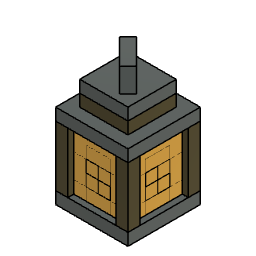
MinecraftMiniLaterne (Autodesk Fusion 360 design; units mm, degrees)
Autodesk Fusion 360 part; units mm, degrees
sketch "Skizze1" plane through (0, 0, 0) normal (0, 0, 1) x (1, 0, 0)
  line L0 (0, 0) -> (60, 0)
  line L1 (60, 0) -> (60, 60)
  line L2 (60, 60) -> (0, 60)
  line L3 (0, 60) -> (0, 0)
  line L4 (0, 0) -> (10, 0)
  line L5 (10, 0) -> (10, 10)
  line L6 (10, 10) -> (0, 10)
  line L7 (0, 10) -> (0, 0)
  line L8 (0, 60) -> (60, 0) construction
  line L9 (60, 60) -> (30, 30) construction
  line L10 (30, 30) -> (0, 0) construction
  line L11 (60, 0) -> (60, 10)
  line L12 (60, 10) -> (50, 10)
  line L13 (50, 10) -> (50, 0)
  line L14 (50, 0) -> (60, 0)
  line L15 (60, 60) -> (50, 60)
  line L16 (50, 60) -> (50, 50)
  line L17 (50, 50) -> (60, 50)
  line L18 (60, 50) -> (60, 60)
  line L19 (0, 60) -> (0, 50)
  line L20 (0, 50) -> (10, 50)
  line L21 (10, 50) -> (10, 60)
  line L22 (10, 60) -> (0, 60)
  line L23 (10, 50) -> (50, 50)
  line L24 (50, 50) -> (50, 10)
  line L25 (50, 10) -> (10, 10)
  line L26 (10, 10) -> (10, 50)
  line L27 (10, 10) -> (7, 10) construction
  line L28 (7, 10) -> (5, 10)
  line L29 (5, 10) -> (5, 50)
  line L30 (5, 50) -> (7, 50)
  line L31 (7, 50) -> (7, 10)
  line L32 (50, 5) -> (10, 5)
  line L33 (10, 5) -> (10, 7)
  line L34 (10, 7) -> (50, 7)
  line L35 (50, 7) -> (50, 5)
  line L36 (55, 50) -> (55, 10)
  line L37 (55, 10) -> (53, 10)
  line L38 (53, 10) -> (53, 50)
  line L39 (53, 50) -> (55, 50)
  line L40 (10, 55) -> (50, 55)
  line L41 (50, 55) -> (50, 53)
  line L42 (50, 53) -> (10, 53)
  line L43 (10, 53) -> (10, 55)
  line L44 (7, 10) -> (5, 10)
  line L45 (5, 10) -> (5, 8)
  line L46 (5, 8) -> (7, 8)
  line L47 (7, 8) -> (7, 10)
  line L48 (10, 7) -> (8, 7)
  line L49 (8, 7) -> (8, 5)
  line L50 (8, 5) -> (10, 5)
  line L51 (10, 5) -> (10, 7)
  line L52 (53, 10) -> (53, 8)
  line L53 (55, 8) -> (55, 10)
  line L54 (55, 10) -> (53, 10)
  line L55 (53, 8) -> (55, 8)
  line L56 (50, 7) -> (50, 5)
  line L57 (50, 5) -> (52, 5)
  line L58 (52, 7) -> (50, 7)
  line L59 (52, 5) -> (52, 7)
  line L60 (50, 53) -> (52, 53)
  line L61 (52, 55) -> (50, 55)
  line L62 (50, 55) -> (50, 53)
  line L63 (52, 53) -> (52, 55)
  line L64 (53, 50) -> (55, 50)
  line L65 (55, 50) -> (55, 52)
  line L66 (53, 52) -> (53, 50)
  line L67 (55, 52) -> (53, 52)
  line L68 (7, 50) -> (7, 52)
  line L69 (5, 52) -> (5, 50)
  line L70 (5, 50) -> (7, 50)
  line L71 (7, 52) -> (5, 52)
  line L72 (10, 53) -> (10, 55)
  line L73 (10, 55) -> (8, 55)
  line L74 (8, 53) -> (10, 53)
  line L75 (8, 55) -> (8, 53)
  line L76 (0, 10) -> (10, 0) construction
  line L77 (7, 3) -> (3, 3)
  line L78 (3, 3) -> (3, 7)
  line L79 (3, 7) -> (7, 7)
  line L80 (7, 7) -> (7, 3)
  line L81 (7, 3) -> (3, 7) construction
  line L82 (3, 3) -> (7, 7) construction
  line L83 (57, 7) -> (57, 3)
  line L84 (57, 3) -> (53, 3)
  line L85 (53, 7) -> (57, 7)
  line L86 (53, 3) -> (53, 7)
  line L87 (53, 57) -> (57, 57)
  line L88 (57, 57) -> (57, 53)
  line L89 (53, 53) -> (53, 57)
  line L90 (57, 53) -> (53, 53)
  line L91 (3, 53) -> (3, 57)
  line L92 (3, 57) -> (7, 57)
  line L93 (7, 53) -> (3, 53)
  line L94 (7, 57) -> (7, 53)
  line L95 (2.8, 7.2) -> (7.2, 7.2)
  line L96 (7.2, 7.2) -> (7.2, 2.8)
  line L97 (7.2, 2.8) -> (2.8, 2.8)
  line L98 (2.8, 2.8) -> (2.8, 7.2)
  line L99 (57.2, 2.8) -> (52.8, 2.8)
  line L100 (52.8, 2.8) -> (52.8, 7.2)
  line L101 (57.2, 7.2) -> (57.2, 2.8)
  line L102 (52.8, 7.2) -> (57.2, 7.2)
  line L103 (57.2, 57.2) -> (57.2, 52.8)
  line L104 (57.2, 52.8) -> (52.8, 52.8)
  line L105 (52.8, 57.2) -> (57.2, 57.2)
  line L106 (52.8, 52.8) -> (52.8, 57.2)
  line L107 (2.8, 57.2) -> (7.2, 57.2)
  line L108 (7.2, 57.2) -> (7.2, 52.8)
  line L109 (2.8, 52.8) -> (2.8, 57.2)
  line L110 (7.2, 52.8) -> (2.8, 52.8)
  point P0 (5, 5)
  dimension "d1" = 60
  dimension "d2" = 60
  dimension "d3" = 10
  dimension "d4" = 10
  dimension "d9" = 360
  dimension "d10" = 3
  dimension "d11" = 2
  dimension "d13" = 360
  dimension "d54" = 2
  dimension "d55" = 2
  dimension "d56" = 2
  dimension "d57" = 2
  dimension "d113" = 4
  dimension "d114" = 4
  dimension "d122" = -0.2
  constraint horizontal L0
  constraint vertical L1
  constraint horizontal L2
  constraint vertical L3
  constraint coincident L0.start L3.end
  constraint horizontal L4
  constraint vertical L5
  constraint horizontal L6
  constraint vertical L7
  constraint midpoint L8 L9.end
  constraint horizontal L23
  constraint vertical L24
  constraint horizontal L25
  constraint vertical L26
  constraint perpendicular L5 L27
  constraint horizontal L28
  constraint vertical L29
  constraint horizontal L30
  constraint vertical L31
  constraint coincident L20 L29.end
  constraint horizontal L44
  constraint vertical L45
  constraint horizontal L46
  constraint vertical L47
  constraint horizontal L48
  constraint vertical L49
  constraint horizontal L50
  constraint vertical L51
  constraint horizontal L77
  constraint perpendicular L77 L78
  constraint parallel L77 L79
  constraint parallel L78 L80
  constraint coincident L81 P0
  constraint coincident L82 P0
  constraint midpoint L76 P0
  measures "d1" distance of L0.start L0.end
  measures "d2" distance of L0.start L2.end
  measures "d3" distance of L0.start L4.end
  measures "d4" distance of L0.start L6.end
  measures "d10" distance of L5.end L27.end
  measures "d11" distance of L27.end L28.end
  measures "d54" distance of L27.end L46.end
  measures "d55" distance of L45.end L46.end
  measures "d56" distance of L33.end L48.end
  measures "d57" distance of L33.end L32.end
  measures "d113" distance of L78.end L79.end
  measures "d114" distance of L77.end L78.end
ref_plane "Arbeitsebene1" through (30, 0, 0) normal (1, 0, 0) x (0, 1, 0)
sketch "Skizze3" plane through (30, 0, 0) normal (1, 0, 0) x (0, 1, 0)
  line L0 (0, 0) -> (60, 0)
  line L1 (30, 0) -> (30, 100) construction
  point P0 (30, 0)
  dimension "d92" = 100
  constraint coincident P0 L1.start
  constraint perpendicular L0 L1
  measures "d92" distance of P0 L1.end
sketch "Skizze2" plane through (0, 0, 0) normal (1, 0, 0) x (0, 1, 0)
  line L0 (0, 0) -> (60, 0)
  line L1 (60, 0) -> (60, 10)
  line L2 (60, 10) -> (0, 10)
  line L3 (0, 10) -> (0, 0)
  line L4 (0, 10) -> (10, 10)
  line L5 (10, 10) -> (10, 60)
  line L6 (10, 60) -> (0, 60)
  line L7 (0, 60) -> (0, 10)
  line L8 (0, 60) -> (60, 60)
  line L9 (60, 60) -> (60, 70)
  line L10 (60, 70) -> (0, 70)
  line L11 (0, 70) -> (0, 60)
  line L12 (60, 10) -> (50, 10)
  line L13 (50, 10) -> (50, 60)
  line L14 (50, 60) -> (60, 60)
  line L15 (60, 60) -> (60, 10)
  line L16 (50, 60) -> (52, 60) construction
  line L17 (52, 60) -> (52, 62) construction
  line L18 (52, 62) -> (50, 62) construction
  line L19 (50, 62) -> (50, 60) construction
  line L20 (10, 10) -> (8, 10) construction
  line L21 (8, 10) -> (8, 8) construction
  line L22 (8, 8) -> (10, 8) construction
  line L23 (10, 8) -> (10, 10) construction
  line L24 (8, 8) -> (52, 8)
  line L25 (52, 8) -> (52, 62)
  line L26 (52, 62) -> (8, 62)
  line L27 (8, 62) -> (8, 8)
  line L28 (50, 10) -> (40, 10)
  line L29 (40, 10) -> (40, 20)
  line L30 (40, 20) -> (50, 20)
  line L31 (50, 20) -> (50, 10)
  line L32 (40, 20) -> (30, 20)
  line L33 (30, 20) -> (30, 30)
  line L34 (30, 30) -> (40, 30)
  line L35 (40, 30) -> (40, 20)
  line L36 (30, 20) -> (20, 20)
  line L37 (20, 20) -> (20, 10)
  line L38 (20, 10) -> (30, 10)
  line L39 (30, 10) -> (30, 20)
  line L40 (20, 20) -> (10, 20)
  line L41 (10, 20) -> (10, 30)
  line L42 (10, 30) -> (20, 30)
  line L43 (20, 30) -> (20, 20)
  line L44 (40, 30) -> (50, 30)
  line L45 (50, 30) -> (50, 40)
  line L46 (50, 40) -> (40, 40)
  line L47 (40, 40) -> (40, 30)
  line L48 (20, 30) -> (30, 30)
  line L49 (30, 30) -> (30, 40)
  line L50 (30, 40) -> (20, 40)
  line L51 (20, 40) -> (20, 30)
  line L52 (40, 40) -> (30, 40)
  line L53 (30, 40) -> (30, 50)
  line L54 (30, 50) -> (40, 50)
  line L55 (40, 50) -> (40, 40)
  line L56 (20, 40) -> (10, 40)
  line L57 (10, 40) -> (10, 50)
  line L58 (10, 50) -> (20, 50)
  line L59 (20, 50) -> (20, 40)
  line L60 (40, 50) -> (50, 50)
  line L61 (50, 50) -> (50, 60)
  line L62 (50, 60) -> (40, 60)
  line L63 (40, 60) -> (40, 50)
  line L64 (20, 50) -> (30, 50)
  line L65 (30, 50) -> (30, 60)
  line L66 (30, 60) -> (20, 60)
  line L67 (20, 60) -> (20, 50)
  line L68 (0, 70) -> (10, 70) construction
  line L69 (10, 70) -> (50, 70)
  line L70 (50, 70) -> (50, 80)
  line L71 (50, 80) -> (10, 80)
  line L72 (10, 80) -> (10, 70)
  line L73 (10, 80) -> (50, 80)
  line L74 (50, 80) -> (50, 90)
  line L75 (50, 90) -> (10, 90)
  line L76 (10, 90) -> (10, 80)
  line L77 (51.58, 61.58) -> (8.42, 61.58)
  line L78 (8.42, 61.58) -> (8.42, 8.42)
  line L79 (8.42, 8.42) -> (51.58, 8.42)
  line L80 (51.58, 8.42) -> (51.58, 61.58)
  dimension "d14" = 60
  dimension "d15" = 10
  dimension "d16" = 10
  dimension "d17" = 50
  dimension "d18" = 60
  dimension "d19" = 10
  dimension "d20" = 10
  dimension "d21" = 2
  dimension "d22" = 2
  dimension "d23" = 2
  dimension "d24" = 2
  dimension "d25" = 10
  dimension "d26" = 10
  dimension "d27" = 10
  dimension "d28" = 10
  dimension "d29" = 10
  dimension "d30" = 10
  dimension "d31" = 10
  dimension "d32" = 10
  dimension "d33" = 10
  dimension "d34" = 10
  dimension "d35" = 10
  dimension "d36" = 10
  dimension "d37" = 10
  dimension "d38" = 10
  dimension "d39" = 10
  dimension "d40" = 10
  dimension "d41" = 10
  dimension "d42" = 10
  dimension "d43" = 10
  dimension "d44" = 10
  dimension "d45" = 10
  dimension "d46" = 40
  dimension "d47" = 10
  dimension "d48" = 40
  dimension "d49" = 10
  dimension "d112" = -0.42
  constraint horizontal L0
  constraint vertical L1
  constraint horizontal L2
  constraint vertical L3
  constraint coincident L0.start L3.end
  constraint horizontal L4
  constraint vertical L5
  constraint horizontal L6
  constraint vertical L7
  constraint horizontal L8
  constraint vertical L9
  constraint horizontal L10
  constraint vertical L11
  constraint horizontal L12
  constraint vertical L13
  constraint horizontal L14
  constraint vertical L15
  constraint horizontal L16
  constraint vertical L17
  constraint horizontal L18
  constraint vertical L19
  constraint horizontal L20
  constraint vertical L21
  constraint horizontal L22
  constraint vertical L23
  constraint horizontal L24
  constraint vertical L25
  constraint horizontal L26
  constraint vertical L27
  constraint horizontal L28
  constraint vertical L29
  constraint horizontal L30
  constraint vertical L31
  constraint horizontal L32
  constraint vertical L33
  constraint horizontal L34
  constraint vertical L35
  constraint horizontal L36
  constraint vertical L37
  constraint horizontal L38
  constraint vertical L39
  constraint horizontal L40
  constraint vertical L41
  constraint horizontal L42
  constraint vertical L43
  constraint horizontal L44
  constraint vertical L45
  constraint horizontal L46
  constraint vertical L47
  constraint horizontal L48
  constraint vertical L49
  constraint horizontal L50
  constraint vertical L51
  constraint horizontal L52
  constraint vertical L53
  constraint horizontal L54
  constraint vertical L55
  constraint horizontal L56
  constraint vertical L57
  constraint horizontal L58
  constraint vertical L59
  constraint horizontal L60
  constraint vertical L61
  constraint horizontal L62
  constraint vertical L63
  constraint horizontal L64
  constraint vertical L65
  constraint horizontal L66
  constraint vertical L67
  constraint coincident L10 L68.end
  constraint horizontal L69
  constraint vertical L70
  constraint horizontal L71
  constraint vertical L72
  constraint horizontal L73
  constraint vertical L74
  constraint horizontal L75
  constraint vertical L76
  measures "d14" distance of L0.start L0.end
  measures "d15" distance of L0.start L2.end
  measures "d16" distance of L2.end L4.end
  measures "d17" distance of L2.end L6.end
  measures "d18" distance of L6.end L8.end
  measures "d19" distance of L6.end L10.end
  measures "d20" distance of L1.end L12.end
  measures "d21" distance of L13.end L16.end
  measures "d22" distance of L13.end L18.end
  measures "d23" distance of L4.end L20.end
  measures "d24" distance of L4.end L22.end
  measures "d25" distance of L12.end L28.end
  measures "d26" distance of L12.end L30.end
  measures "d27" distance of L29.end L32.end
  measures "d28" distance of L29.end L34.end
  measures "d29" distance of L32.end L36.end
  measures "d30" distance of L32.end L38.end
  measures "d31" distance of L36.end L40.end
  measures "d32" distance of L36.end L42.end
  measures "d33" distance of L34.end L44.end
  measures "d34" distance of L34.end L46.end
  measures "d35" distance of L42.end L33.end
  measures "d36" distance of L42.end L50.end
  measures "d37" distance of L46.end L49.end
  measures "d38" distance of L46.end L54.end
  measures "d39" distance of L50.end L56.end
  measures "d40" distance of L50.end L58.end
  measures "d41" distance of L54.end L60.end
  measures "d42" distance of L54.end L62.end
  measures "d43" distance of L58.end L53.end
  measures "d44" distance of L58.end L66.end
  measures "d45" distance of L10.end L68.end
  measures "d46" distance of L68.end L69.end
  measures "d47" distance of L68.end L71.end
  measures "d48" distance of L71.end L70.end
  measures "d49" distance of L71.end L75.end
extrude "Extrusion1" add sketch "Skizze1" along normal blind 10 contours L0 L3 L4 L5 L6 L7 L45 L46 L47 L48 L49 L50 | L0 L5 L13 L32 | L3 L6 L20 L29 | L0 L1 L11 L12 L13 L14 L52 L53 L55 L57 L58 L59 | L2 L3 L19 L20 L21 L22 L68 L69 L71 L73 L74 L75 | L5 L13 L25 L34 | L6 L20 L26 L31 | L1 L12 L17 L36 | L23 L24 L25 L26 | L2 L16 L21 L40 | L1 L2 L15 L16 L17 L18 L60 L61 L63 L65 L66 L67 | L12 L17 L24 L38 | L16 L21 L23 L42 | L77 L78 L79 L80 | L83 L84 L85 L86 | L87 L88 L89 L90 | L91 L92 L93 L94 | L95 L96 L97 L98 | L99 L100 L101 L102 | L103 L104 L105 L106 | L107 L108 L109 L110 makes body 1
extrude "Extrusion2" add sketch "Skizze1" along normal blind 8 contours L5 L33 L48 L49 L50 L51 | L5 L13 L32 L33 L34 L35 L51 L56 | L6 L20 L28 L29 L30 L31 L44 L70 | L6 L28 L44 L45 L46 L47 | L13 L35 L56 L57 L58 L59 | L20 L30 L68 L69 L70 L71 | L12 L37 L52 L53 L54 L55 | L12 L17 L36 L37 L38 L39 L54 L64 | L16 L21 L40 L41 L42 L43 L62 L72 | L21 L43 L72 L73 L74 L75 | L17 L39 L64 L65 L66 L67 | L16 L41 L60 L61 L62 L63 bodies 1
extrude "Extrusion3" add sketch "Skizze1" along normal blind 50 from surface at 10 separate body contours L0 L3 L4 L5 L6 L7 L45 L46 L47 L48 L49 L50 | L0 L1 L11 L12 L13 L14 L52 L53 L55 L57 L58 L59 | L2 L3 L19 L20 L21 L22 L68 L69 L71 L73 L74 L75 | L1 L2 L15 L16 L17 L18 L60 L61 L63 L65 L66 L67 | L77 L78 L79 L80 | L83 L84 L85 L86 | L87 L88 L89 L90 | L91 L92 L93 L94 | L95 L96 L97 L98 | L99 L100 L101 L102 | L103 L104 L105 L106 | L107 L108 L109 L110 makes body 2 at (0, 6.6667, 26.6667) makes body 3 at (6.6667, 60, 26.6667) makes body 4 at (60, 3.3333, 26.6667) makes body 5 at (56.6667, 60, 26.6667)
extrude "Extrusion18" add sketch "Skizze1" along normal blind 5 from surface at 60 contours L77 L78 L79 L80 | L83 L84 L85 L86 | L87 L88 L89 L90 | L91 L92 L93 L94 bodies 2 3 4 5
extrude "Extrusion4" add sketch "Skizze1" along normal blind 10 from surface at 60 separate body contours L0 L3 L4 L5 L6 L7 L45 L46 L47 L48 L49 L50 | L0 L5 L13 L32 | L3 L6 L20 L29 | L0 L1 L11 L12 L13 L14 L52 L53 L55 L57 L58 L59 | L2 L3 L19 L20 L21 L22 L68 L69 L71 L73 L74 L75 | L5 L13 L25 L34 | L6 L20 L26 L31 | L1 L12 L17 L36 | L23 L24 L25 L26 | L2 L16 L21 L40 | L1 L2 L15 L16 L17 L18 L60 L61 L63 L65 L66 L67 | L12 L17 L24 L38 | L16 L21 L23 L42 | L77 L78 L79 L80 | L83 L84 L85 L86 | L87 L88 L89 L90 | L91 L92 L93 L94 | L95 L96 L97 L98 | L99 L100 L101 L102 | L103 L104 L105 L106 | L107 L108 L109 L110 makes body 6
extrude "Extrusion19" cut sketch "Skizze1" along normal blind 7 from surface at 60 contours L77 L78 L79 L80 | L83 L84 L85 L86 | L87 L88 L89 L90 | L91 L92 L93 L94 | L95 L96 L97 L98 | L99 L100 L101 L102 | L103 L104 L105 L106 | L107 L108 L109 L110 bodies 6
extrude "Extrusion5" add sketch "Skizze1" against normal blind 8 from surface at 70 contours L5 L33 L48 L49 L50 L51 | L5 L13 L32 L33 L34 L35 L51 L56 | L6 L20 L28 L29 L30 L31 L44 L70 | L6 L28 L44 L45 L46 L47 | L13 L35 L56 L57 L58 L59 | L20 L30 L68 L69 L70 L71 | L12 L37 L52 L53 L54 L55 | L12 L17 L36 L37 L38 L39 L54 L64 | L16 L21 L40 L41 L42 L43 L62 L72 | L21 L43 L72 L73 L74 L75 | L17 L39 L64 L65 L66 L67 | L16 L41 L60 L61 L62 L63 bodies 6
extrude "Extrusion6" add sketch "Skizze2" along normal blind 40 from surface at 10 separate body contours L10 L69 L70 L71 L72 L73 makes body 7
extrude "Extrusion7" add sketch "Skizze2" along normal blind 40 from surface at 10 separate body contours L71 L73 L74 L75 L76 makes body 8
extrude "Extrusion8" add sketch "Skizze2" against normal blind 1.8 from surface at 7 separate body contours L2 L4 L5 L6 L8 L41 L57 L78 | L2 L4 L12 L28 L38 L78 L79 L80 | L2 L8 L12 L13 L14 L31 L45 L61 L80 | L6 L8 L14 L62 L66 L77 L78 L80 makes body 9
extrude "Extrusion9" add sketch "Skizze2" along normal blind 0.4 from surface at 5.2 separate body contours L32 L33 L34 L35 | L48 L49 L50 L51 makes body 10 at (5.2, 23.3333, 36.6667)
extrude "Extrusion10" add sketch "Skizze2" along normal blind 0.2 from surface at 5.2 contours L33 L36 L43 L48 | L34 L47 L49 L52 bodies 10
extrude "Extrusion11" add sketch "Skizze2" along normal blind 0.6 from surface at 5.2 contours L2 L36 L37 L38 L39 | L5 L40 L41 L42 L43 | L2 L29 L32 L39 | L13 L30 L35 L44 | L5 L42 L51 L56 | L13 L44 L45 L46 L47 | L50 L53 L59 L64 | L52 L53 L54 L55 bodies 9 10
extrude "Extrusion12" add sketch "Skizze2" along normal blind 0.8 from surface at 5.2 contours L2 L5 L37 L40 | L2 L13 L28 L29 L30 L31 | L5 L56 L57 L58 L59 | L8 L64 L65 L66 L67 | L8 L54 L63 L65 | L13 L46 L55 L60 bodies 9
extrude "Extrusion13" add sketch "Skizze2" along normal blind 1 from surface at 5.2 contours L5 L8 L58 L67 | L8 L13 L60 L61 L62 L63 bodies 9
pattern_circular "C-Anordnung1" count 4 over 360 about axis through (30, 30, 0) along (0, 0, 1) of bodies 9 makes body 11 at (22.8067, 5.2, 26.14) makes body 12 at (54.8, 22.8067, 26.14) makes body 13 at (37.1933, 54.8, 26.14)
sketch "Skizze4" plane through (0, 0, 90) normal (0, 0, 1) x (-1, 0, 0)
  line L0 (-10, -50) -> (-10, -10)
  line L1 (-10, -10) -> (-50, -10)
  line L2 (-50, -10) -> (-50, -50)
  line L3 (-50, -50) -> (-10, -50)
  line L4 (-50, -10) -> (-10, -50) construction
  line L5 (-10, -10) -> (-30, -30) construction
  line L6 (-30, -37.0711) -> (-37.0711, -30)
  line L7 (-37.0711, -30) -> (-30, -22.9289)
  line L8 (-30, -22.9289) -> (-22.9289, -30)
  line L9 (-22.9289, -30) -> (-30, -37.0711)
  line L10 (-30, -37.0711) -> (-30, -22.9289) construction
  line L11 (-37.0711, -30) -> (-22.9289, -30) construction
  line L12 (-30, -37.0711) -> (-22.9289, -30)
  line L13 (-22.9289, -30) -> (-15.8579, -37.0711)
  line L14 (-15.8579, -37.0711) -> (-22.9289, -44.1421)
  line L15 (-22.9289, -44.1421) -> (-30, -37.0711)
  line L16 (-37.0711, -30) -> (-30, -22.9289)
  line L17 (-30, -22.9289) -> (-37.0711, -15.8579)
  line L18 (-37.0711, -15.8579) -> (-44.1421, -22.9289)
  line L19 (-44.1421, -22.9289) -> (-37.0711, -30)
  point P0 (-30, -30)
  dimension "d95" = 10
  dimension "d96" = 10
  dimension "d97" = 10
  dimension "d98" = 10
  constraint coincident L1.end L2.start
  constraint coincident L0.start L3.end
  constraint coincident L0.end L1.start
  constraint midpoint L4 P0
  constraint perpendicular L6 L7
  constraint parallel L6 L8
  constraint parallel L7 L9
  constraint coincident L10 P0
  constraint coincident L11 P0
  constraint coincident P0 L5.end
  constraint perpendicular L12 L13
  constraint parallel L12 L14
  constraint parallel L13 L15
  constraint perpendicular L16 L17
  constraint parallel L16 L18
  constraint parallel L17 L19
  measures "d95" distance of L7.end L8.end
  measures "d96" distance of L6.end L7.end
  measures "d97" distance of L6.start L14.end
  measures "d98" distance of L6.end L18.end
extrude "Extrusion14" add sketch "Skizze4" along normal blind 10 separate body contours L9 L12 L13 L14 L15 | L7 L16 L17 L18 L19 makes body 14 at (39.4281, 27.643, 96.6667) makes body 15 at (18.2149, 39.4281, 93.3333)
extrude "Extrusion15" add sketch "Skizze4" along normal blind 10 from surface at 10 contours L6 L7 L8 L9 L12 L16 | L9 L12 L13 L14 L15 | L7 L16 L17 L18 L19 bodies 14 15
sketch "Skizze5" plane through (0, 0, 0) normal (0, 0, -1) x (1, 0, 0)
  line L0 (0, -60) -> (60, -60)
  line L1 (60, -60) -> (60, 0)
  line L2 (60, 0) -> (0, 0)
  line L3 (0, 0) -> (0, -60)
  line L4 (0, 0) -> (60, -60) construction
  line L5 (60, 0) -> (30, -30) construction
  circle A0 centre (30, -30) radius 17.1
  line L6 (30, -30) -> (45.5, -30) construction
  circle A1 centre (45.5, -30) radius 1.2
  circle A2 centre (45.5, -30) radius 2.4
  line L7 (45.5, -30) -> (45.5, -32.4) construction
  line L8 (45.5, -32.4) -> (46.9307, -32.4)
  line L9 (45.5, -27.6) -> (46.9307, -27.6)
  line L10 (30, -30) -> (30, -39.5) construction
  circle A3 centre (14.5, -30) radius 2.4
  circle A4 centre (14.5, -30) radius 1.2
  line L11 (14.5, -32.4) -> (13.0693, -32.4)
  line L12 (14.5, -27.6) -> (13.0693, -27.6)
  dimension "d104" = 34.2
  dimension "d105" = 15.5
  dimension "d106" = 2.4
  dimension "d107" = 4.8
  constraint coincident L2.end L3.start
  constraint coincident L0.end L1.start
  constraint coincident L1.end L2.start
  constraint midpoint L4 L5.end
  constraint coincident L5.end A0.centre
  constraint horizontal L6
  constraint coincident L6.end A1.centre
  constraint concentric A1 A2
  constraint coincident A2 L7.end
  constraint perpendicular L6 L7
  constraint coincident A0 L8.end
  constraint tangent A2 L8
  constraint symmetric L6 L7.end L9.start
  constraint symmetric L6 L8.end L9.end
  constraint perpendicular L6 L10
  constraint symmetric A1 L10 A4
  constraint symmetric A2 L10 A3
  constraint symmetric L7.end L10 L11.start
  constraint symmetric L8.end L10 L11.end
  constraint symmetric L9.start L10 L12.start
  constraint symmetric L9.end L10 L12.end
  measures "d104" diameter of A0
  measures "d105" distance of L5.end L6.end
  measures "d106" diameter of A1
  measures "d107" diameter of A2
extrude "Extrusion16" cut sketch "Skizze5" against normal blind 10 contours A0 A2 L8 L9 A3 L11 L12 | A1 | A4 bodies 1
extrude "Extrusion17" cut sketch "Skizze5" against normal blind 3 contours A0 A2 L9 | A0 A3 L12 | A0 A2 | A0 A3 | A0 A2 L8 | A0 A3 L11 picked at (46.6285, -28.5495) picked at (13.1783, -28.8937) bodies 1
chamfer "Fase1" distance 1 angle 45 4 faces at (55.6667, 54.3333, 65) (54.3333, 5.6667, 65) (4.3333, 54.3333, 65) (5.6667, 4.3333, 65) on bodies 2 3 4 5
equation "d1 = 6 * pixel"
equation "d2 = d1"
equation "d3 = pixel"
equation "d4 = pixel"
equation "pixel = 10 mm"
equation "linienhöhe = 0.2 mm"
equation "linienbreite = 0.42 mm"
equation "d10 = 0.3 * pixel"
equation "d11 = 0.2 * pixel"
equation "d14 = d1"
equation "d15 = pixel"
equation "d16 = pixel"
equation "d17 = pixel * 5"
equation "d18 = d1"
equation "d19 = pixel"
equation "d20 = pixel"
equation "d21 = pixel * 0.2"
equation "d22 = d21"
equation "d23 = d21"
equation "d24 = d21"
equation "d25 = pixel"
equation "d26 = pixel"
equation "d27 = pixel"
equation "d28 = pixel"
equation "d29 = pixel"
equation "d30 = pixel"
equation "d31 = pixel"
equation "d32 = pixel"
equation "d33 = pixel"
equation "d34 = pixel"
equation "d35 = pixel"
equation "d36 = pixel"
equation "d37 = pixel"
equation "d38 = pixel"
equation "d39 = pixel"
equation "d40 = pixel"
equation "d41 = pixel"
equation "d42 = pixel"
equation "d43 = pixel"
equation "d44 = pixel"
equation "d45 = pixel"
equation "d46 = pixel * 4"
equation "d47 = pixel"
equation "d48 = pixel * 4"
equation "d49 = pixel"
equation "d50 = pixel"
equation "d52 = pixel - pixel * 0.2"
equation "d54 = pixel * 0.2"
equation "d55 = d11"
equation "d56 = d54"
equation "d57 = d11"
equation "d59 = pixel * 5"
equation "d62 = pixel"
equation "d65 = -( pixel - pixel * 0.2 )"
equation "d67 = pixel"
equation "d68 = 4 * pixel"
equation "d71 = pixel * 4"
equation "d74 = -( pixel * 0.18 )"
equation "d77 = linienhöhe * 2"
equation "d80 = linienhöhe"
equation "d83 = linienhöhe * 3"
equation "d86 = linienhöhe * 4"
equation "d89 = linienhöhe * 5"
equation "d91 = pixel * 3"
equation "d95 = pixel"
equation "d96 = pixel"
equation "d97 = pixel"
equation "d98 = pixel"
equation "d99 = pixel"
equation "d102 = pixel"
equation "d105 = ( 31 / 2 ) * 1 mm"
equation "d113 = pixel * 0.4"
equation "d114 = pixel * 0.4"
equation "d116 = pixel * 0.5"
equation "d119 = pixel * 0.7"
named bodies: "bottom", "stick1", "stick2", "stick3", "stick4", "top1", "top2", "top3", "plate1", "plate2", "plate3", "plate4", "handle"
